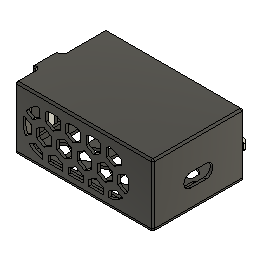
ESP32Case (Autodesk Fusion 360 design; units mm, degrees)
Autodesk Fusion 360 part; units mm, degrees
(part 1 of 3)
sketch "Skizze1" plane through (0, 0, 0) normal (0, 0, 1) x (1, 0, 0)
  line L0 (0, 0) -> (72, 0)
  line L1 (72, 0) -> (72, 49.5)
  line L2 (72, 49.5) -> (0, 49.5)
  line L3 (0, 49.5) -> (0, 0)
  dimension "d1" = 72
  dimension "d2" = 49.5
  constraint horizontal L0
  constraint vertical L1
  constraint horizontal L2
  constraint vertical L3
  constraint coincident L0.start L3.end
  measures "d1" distance of L0.start L0.end
  measures "d2" distance of L0.start L2.end
extrude "Extrusion1" add sketch "Skizze1" along normal blind 1.4 makes body 1
sketch "Skizze2" plane through (0, 0, 0) normal (0, 0, -1) x (1, 0, 0)
  line L0 (0, 0) -> (0, -49.5)
  line L1 (0, -49.5) -> (72, -49.5)
  line L2 (72, -49.5) -> (72, 0)
  line L3 (72, 0) -> (0, 0)
  line L4 (-2, -51.5) -> (74, -51.5)
  line L5 (74, -51.5) -> (74, 2)
  line L6 (74, 2) -> (-2, 2)
  line L7 (-2, 2) -> (-2, -51.5)
  line L8 (0, 0) -> (72, 0)
  line L9 (72, 0) -> (72, -4)
  line L10 (72, -4) -> (0, -4)
  line L11 (0, -4) -> (0, 0)
  line L12 (0, -49.5) -> (72, -49.5)
  line L13 (72, -49.5) -> (72, -45.5)
  line L14 (72, -45.5) -> (0, -45.5)
  line L15 (0, -45.5) -> (0, -49.5)
  line L16 (0, -49.5) -> (19, -49.5)
  line L17 (19, -49.5) -> (19, -45.5)
  line L18 (19, -45.5) -> (0, -45.5)
  line L19 (0, -45.5) -> (0, -49.5)
  line L20 (19, -45.5) -> (31, -45.5)
  line L21 (31, -45.5) -> (31, -49.5)
  line L22 (31, -49.5) -> (19, -49.5)
  line L23 (19, -49.5) -> (19, -45.5)
  line L24 (72, 0) -> (77, 0)
  line L25 (77, 0) -> (77, -49.5)
  line L26 (77, -49.5) -> (72, -49.5)
  line L27 (72, -49.5) -> (72, 0)
  line L28 (72, 2) -> (79, 2)
  line L29 (79, 2) -> (79, -51.5)
  line L30 (79, -51.5) -> (72, -51.5)
  dimension "d5" = 2
  dimension "d6" = 4
  dimension "d7" = 19
  dimension "d8" = 12
  dimension "d9" = 5
  dimension "d10" = -2
  constraint horizontal L8
  constraint vertical L9
  constraint horizontal L10
  constraint vertical L11
  constraint coincident L2 L9.end
  constraint coincident L0.start L3.end
  constraint horizontal L12
  constraint vertical L13
  constraint horizontal L14
  constraint vertical L15
  constraint coincident L0.end L1.start
  constraint horizontal L16
  constraint vertical L17
  constraint horizontal L18
  constraint vertical L19
  constraint horizontal L20
  constraint vertical L21
  constraint horizontal L22
  constraint vertical L23
  constraint horizontal L24
  constraint vertical L25
  constraint horizontal L26
  constraint vertical L27
  constraint coincident L2.end L3.start
  measures "d6" distance of L0.end L14.end
  measures "d7" distance of L0.end L16.end
  measures "d8" distance of L17.end L20.end
  measures "d9" distance of L2.end L24.end
extrude "Extrusion2" add sketch "Skizze2" along normal blind 2 separate body contours L0 L2 L3 L8 L9 L10 L11 L27 | L0 L1 L3 L4 L5 L6 L7 L8 L11 L12 L15 L16 L19 L22 L24 L26 L28 L30 | L2 L5 L9 L13 L24 L26 L27 | L0 L1 L12 L14 L15 L16 L17 L18 L19 L23 | L5 L24 L25 L26 | L5 L24 L25 L26 L28 L29 L30 | L1 L2 L12 L13 L14 L21 L27 makes body 2
sketch "Skizze3" plane through (0, 0, 0) normal (0, 0, 1) x (-1, 0, 0)
  line L0 (-72, -4) -> (0, -4)
  line L1 (0, -4) -> (0, -45.5)
  line L2 (0, -45.5) -> (-19, -45.5)
  line L3 (-19, -45.5) -> (-19, -49.5)
  line L4 (-19, -49.5) -> (-31, -49.5)
  line L5 (-31, -49.5) -> (-31, -45.5)
  line L6 (-31, -45.5) -> (-72, -45.5)
  line L7 (-72, -45.5) -> (-72, -4)
  line L8 (2, 2) -> (-79, 2)
  line L9 (-79, 2) -> (-79, -51.5)
  line L10 (-79, -51.5) -> (2, -51.5)
  line L11 (2, -51.5) -> (2, 2)
extrude "Extrusion3" add sketch "Skizze3" along normal blind 2 contours L0 L1 L2 L3 L4 L5 L6 L7 | L8 L9 L10 L11 bodies 2
move_body "Verschieben1" bodies 1 to x (1, 0, 0) y (0, 1, 0) z (0, 0, 1) at (0, 0, -3.4)
sketch "Skizze4" plane through (0, 0, -2) normal (0, 0, -1) x (1, 0, 0)
  line L0 (0, -4) -> (72, -4)
  line L1 (72, -4) -> (72, -45.5)
  line L2 (72, -45.5) -> (31, -45.5)
  line L3 (31, -45.5) -> (31, -49.5)
  line L4 (31, -49.5) -> (19, -49.5)
  line L5 (19, -49.5) -> (19, -45.5)
  line L6 (19, -45.5) -> (0, -45.5)
  line L7 (0, -45.5) -> (0, -4)
  line L8 (79, 2) -> (-2, 2)
  line L9 (-2, 2) -> (-2, -51.5)
  line L10 (-2, -51.5) -> (79, -51.5)
  line L11 (79, -51.5) -> (79, 2)
  line L12 (-0.5, -50) -> (77.5, -50)
  line L13 (77.5, -50) -> (77.5, 0.5)
  line L14 (77.5, 0.5) -> (-0.5, 0.5)
  line L15 (-0.5, 0.5) -> (-0.5, -50)
  line L16 (72, -4) -> (72, 0.5)
  line L17 (72, -45.5) -> (72, -50)
  line L18 (72, 0.5) -> (73.5, 0.5)
  line L19 (73.5, 0.5) -> (73.5, -50)
  line L20 (73.5, -50) -> (72, -50)
  line L21 (72, -50) -> (72, 0.5)
  dimension "d15" = -1.5
  dimension "d16" = 1.5
  constraint coincident L0.end L1.start
  constraint coincident L14 L16.end
  constraint perpendicular L14 L16
  constraint coincident L1.end L2.start
  constraint coincident L12 L17.end
  constraint perpendicular L12 L17
  constraint horizontal L18
  constraint vertical L19
  constraint horizontal L20
  constraint vertical L21
  measures "d16" distance of L16.end L18.end
extrude "Extrusion4" add sketch "Skizze4" along normal blind 31 bodies 2
extrude "Extrusion5" add sketch "Skizze4" along normal blind 12.4 contours L1 L12 L14 L16 L17 L18 L19 L20 L21 bodies 2
extrude "Extrusion6" add sketch "Skizze4" along normal blind 12.4 contours L12 L13 L14 L19 bodies 2
sketch "Skizze5" plane through (0, 0, -33) normal (0, 0, -1) x (1, 0, 0)
  line L0 (77.5, 0.5) -> (77.5, -50)
  line L1 (77.5, -50) -> (-0.5, -50)
  line L2 (-0.5, -50) -> (-0.5, 0.5)
  line L3 (-0.5, 0.5) -> (77.5, 0.5)
  line L4 (79, -51.5) -> (79, 2)
  line L5 (79, 2) -> (-2, 2)
  line L6 (-2, 2) -> (-2, -51.5)
  line L7 (-2, -51.5) -> (79, -51.5)
  line L8 (-2, -15.5) -> (7, -15.5)
  line L9 (0, 0) -> (72, 0)
  line L10 (-2, -21.5) -> (2, -21.5)
  line L11 (-2, -15.5) -> (0, -15.5)
  line L12 (0, -15.5) -> (0, -21.5)
  line L13 (0, -21.5) -> (-2, -21.5)
  line L14 (-2, -21.5) -> (-2, -15.5)
  dimension "d23" = 15.5
  dimension "d24" = 6
  constraint coincident L6 L8.start
  constraint perpendicular L6 L8
  constraint coincident L6 L10.start
  constraint perpendicular L2 L10
  constraint horizontal L11
  constraint vertical L12
  constraint horizontal L13
  constraint vertical L14
  constraint midpoint L10 L12.end
  measures "d23" distance of L8 L9
  measures "d24" distance of L8 L10
extrude "Extrusion7" cut sketch "Skizze5" against normal blind 27 contours L2 L6 L8 L10 L11 L13 L14 bodies 2
sketch "Skizze6" plane through (-2, 0, 0) normal (-1, 0, 0) x (0, -1, 0)
  line L0 (-15.5, -6) -> (-15.5, -33)
  line L1 (-15.5, -33) -> (2, -33)
  line L2 (2, -33) -> (2, 2)
  line L3 (2, 2) -> (-51.5, 2)
  line L4 (-51.5, 2) -> (-51.5, -33)
  line L5 (-51.5, -33) -> (-21.5, -33)
  line L6 (-21.5, -33) -> (-21.5, -6)
  line L7 (-21.5, -6) -> (-15.5, -6)
  line L8 (0, -3.4) -> (-49.5, -3.4)
  line L9 (-49.5, -3.4) -> (0, -3.4)
  circle A0 centre (-18.5, -6.4) radius 3
  constraint tangent L8 A0
  constraint tangent L0 A0
  constraint tangent L6 A0
extrude "Extrusion8" cut sketch "Skizze6" against normal blind 1.5 contours L7 A0 picked at (-17.8417, -5.3806) bodies 2
sketch "Skizze7" plane through (79, 0, 0) normal (1, 0, 0) x (0, 1, 0)
  line L0 (-2, 2) -> (-2, -33)
  line L1 (-2, -33) -> (51.5, -33)
  line L2 (51.5, -33) -> (51.5, 2)
  line L3 (51.5, 2) -> (-2, 2)
  line L4 (50, -14.4) -> (-0.5, -14.4)
  line L5 (-0.5, -14.4) -> (50, -14.4)
  line L6 (48.75, -19) -> (0.75, -19) construction
  line L7 (29.25, -15) -> (20.25, -15)
  arc A0 (20.25, -15) -> (20.25, -23) centre (20.25, -19) ccw
  line L8 (20.25, -23) -> (29.25, -23)
  arc A1 (29.25, -23) -> (29.25, -15) centre (29.25, -19) ccw
  line L9 (29.25, -19) -> (20.25, -19) construction
  point P0 (24.75, -19)
  dimension "d29" = 4.6
  dimension "d30" = 8
  dimension "d31" = 9
  dimension "d32" = 53.5
  dimension "d33" = 26.75
  constraint parallel L4 L6
  constraint tangent L7 A0
  constraint tangent A0 L8
  constraint parallel L7 L8
  constraint tangent L8 A1
  constraint tangent L7 A1
  constraint parallel L6 L9
  constraint midpoint L6 P0
  constraint midpoint L9 P0
  measures "d29" distance of L4 L6
  measures "d30" diameter of A0
  measures "d31" distance of A0.end L8.end
  measures "d32" distance of L0.end L1.end
  measures "d33" distance of L0 P0
extrude "Extrusion9" cut sketch "Skizze7" against normal blind 7 contours L7 A0 L8 A1 bodies 2
sketch "Skizze8" plane through (0, 51.5, 0) normal (0, 1, 0) x (-1, 0, 0)
  line L0 (-79, 2) -> (-79, -33)
  line L1 (-79, -33) -> (2, -33)
  line L2 (2, -33) -> (2, 2)
  line L3 (2, 2) -> (-79, 2)
  line L4 (-72, -14.4) -> (-77.5, -14.4)
  line L5 (-77.5, -15) -> (-79, -15)
  line L6 (-79, -15) -> (-77.5, -15)
  line L7 (-77.5, -14.4) -> (-72, -14.4)
  line L8 (-77.5, -14.4) -> (-70, -14.4)
  line L9 (-70, -14.4) -> (-70, -16)
  line L10 (-70, -16) -> (-77.5, -16)
  line L11 (-77.5, -16) -> (-77.5, -14.4)
  line L12 (-77.5, -16) -> (-71.5, -16)
  line L13 (-71.5, -16) -> (-71.5, -20)
  line L14 (-71.5, -20) -> (-77.5, -20)
  line L15 (-77.5, -20) -> (-77.5, -16)
  line L16 (-79, -14.5) -> (-70, -14.5)
  line L17 (-70, -14.5) -> (-70, -21.5)
  line L18 (-70, -21.5) -> (-79, -21.5)
  line L19 (-79, -21.5) -> (-79, -14.5)
  dimension "d36" = 6
  dimension "d37" = 4
  dimension "d38" = -1.5
  constraint horizontal L8
  constraint vertical L9
  constraint horizontal L10
  constraint vertical L11
  constraint coincident L4.end L7.start
  constraint horizontal L12
  constraint vertical L13
  constraint horizontal L14
  constraint vertical L15
  measures "d36" distance of L10.end L12.end
  measures "d37" distance of L10.end L14.end
extrude "Extrusion10" add sketch "Skizze8" against normal blind 8 contours L0 L5 L6 L11 L16 L19 | L0 L5 L6 L10 L11 L13 L14 L15 L17 L18 L19 | L9 L10 L11 L12 L16 L17 bodies 2
extrude "Extrusion11" add 1 faces at (75, 45.6667, -14.5) along direction (0, 0, 1) blind 0.1 on bodies 2 bodies 2
chamfer "Fase1" distance 2 angle 45 1 edges at (72, 46.75, -14.4) on bodies 2
extrude "Extrusion12" cut 1 faces at (73.5, 50, -18.6667) along direction (0, 1, 0) blind 10 on bodies 2 bodies 2
sketch "Skizze9" plane through (0, 51.5, 0) normal (0, 1, 0) x (-1, 0, 0)
  line L0 (-71.5, -16) -> (-71.5, -20)
  line L1 (-71.5, -20) -> (-77.5, -20)
  line L2 (-77.5, -20) -> (-77.5, -16)
  line L3 (-77.5, -16) -> (-71.5, -16)
  line L4 (-79, 2) -> (-79, -33)
  line L5 (-79, -33) -> (2, -33)
  line L6 (2, -33) -> (2, 2)
  line L7 (2, 2) -> (-79, 2)
  line L8 (-51.9385, -29.7827) -> (-15.9385, -29.7827)
  arc A0 (-15.9385, -29.7827) -> (-15.9385, -3.6265) centre (-15.9385, -16.7046) ccw
  line L9 (-15.9385, -3.6265) -> (-51.9385, -3.6265)
  arc A1 (-51.9385, -3.6265) -> (-51.9385, -29.7827) centre (-51.9385, -16.7046) ccw
  line L10 (-51.9385, -16.7046) -> (-15.9385, -16.7046) construction
  line L11 (0, -3.4) -> (-72, -3.4)
  line L12 (-72, -3.4) -> (0, -3.4)
  line L13 (106.9565, 20) -> (111.2866, 22.5)
  line L14 (111.2866, 22.5) -> (111.2866, 27.5)
  line L15 (111.2866, 27.5) -> (106.9565, 30)
  line L16 (106.9565, 30) -> (102.6264, 27.5)
  line L17 (102.6264, 27.5) -> (102.6264, 22.5)
  line L18 (102.6264, 22.5) -> (106.9565, 20)
  line L19 (106.9565, 30) -> (34, 30)
  line L20 (99.3775, 22.5) -> (99.3775, 27.5)
  line L21 (99.3775, 27.5) -> (95.0474, 30)
  line L22 (95.0474, 30) -> (90.7173, 27.5)
  line L23 (90.7173, 27.5) -> (90.7173, 22.5)
  line L24 (90.7173, 22.5) -> (95.0474, 20)
  line L25 (95.0474, 20) -> (99.3775, 22.5)
  line L26 (87.4684, 22.5) -> (87.4684, 27.5)
  line L27 (87.4684, 27.5) -> (83.1383, 30)
  line L28 (83.1383, 30) -> (78.8082, 27.5)
  line L29 (78.8082, 27.5) -> (78.8082, 22.5)
  line L30 (78.8082, 22.5) -> (83.1383, 20)
  line L31 (83.1383, 20) -> (87.4684, 22.5)
  line L32 (75.5593, 22.5) -> (75.5593, 27.5)
  line L33 (75.5593, 27.5) -> (71.2292, 30)
  line L34 (71.2292, 30) -> (66.8991, 27.5)
  line L35 (66.8991, 27.5) -> (66.8991, 22.5)
  line L36 (66.8991, 22.5) -> (71.2292, 20)
  line L37 (71.2292, 20) -> (75.5593, 22.5)
  line L38 (63.6503, 22.5) -> (63.6503, 27.5)
  line L39 (63.6503, 27.5) -> (59.3201, 30)
  line L40 (59.3201, 30) -> (54.99, 27.5)
  line L41 (54.99, 27.5) -> (54.99, 22.5)
  line L42 (54.99, 22.5) -> (59.3201, 20)
  line L43 (59.3201, 20) -> (63.6503, 22.5)
  line L44 (51.7412, 22.5) -> (51.7412, 27.5)
  line L45 (51.7412, 27.5) -> (47.411, 30)
  line L46 (47.411, 30) -> (43.0809, 27.5)
  line L47 (43.0809, 27.5) -> (43.0809, 22.5)
  line L48 (43.0809, 22.5) -> (47.411, 20)
  line L49 (47.411, 20) -> (51.7412, 22.5)
  line L50 (39.8321, 22.5) -> (39.8321, 27.5)
  line L51 (39.8321, 27.5) -> (35.5019, 30)
  line L52 (35.5019, 30) -> (31.1718, 27.5)
  line L53 (31.1718, 27.5) -> (31.1718, 22.5)
  line L54 (31.1718, 22.5) -> (35.5019, 20)
  line L55 (35.5019, 20) -> (39.8321, 22.5)
  line L56 (27.923, 22.5) -> (27.923, 27.5)
  line L57 (27.923, 27.5) -> (23.5929, 30)
  line L58 (23.5929, 30) -> (19.2627, 27.5)
  line L59 (19.2627, 27.5) -> (19.2627, 22.5)
  line L60 (19.2627, 22.5) -> (23.5929, 20)
  line L61 (23.5929, 20) -> (27.923, 22.5)
  line L62 (16.0139, 22.5) -> (16.0139, 27.5)
  line L63 (16.0139, 27.5) -> (11.6838, 30)
  line L64 (11.6838, 30) -> (7.3536, 27.5)
  line L65 (7.3536, 27.5) -> (7.3536, 22.5)
  line L66 (7.3536, 22.5) -> (11.6838, 20)
  line L67 (11.6838, 20) -> (16.0139, 22.5)
  line L68 (4.1048, 22.5) -> (4.1048, 27.5)
  line L69 (4.1048, 27.5) -> (-0.2253, 30)
  line L70 (-0.2253, 30) -> (-4.5555, 27.5)
  line L71 (-4.5555, 27.5) -> (-4.5555, 22.5)
  line L72 (-4.5555, 22.5) -> (-0.2253, 20)
  line L73 (-0.2253, 20) -> (4.1048, 22.5)
  line L74 (-7.8043, 22.5) -> (-7.8043, 27.5)
  line L75 (-7.8043, 27.5) -> (-12.1344, 30)
  line L76 (-12.1344, 30) -> (-16.4645, 27.5)
  line L77 (-16.4645, 27.5) -> (-16.4645, 22.5)
  line L78 (-16.4645, 22.5) -> (-12.1344, 20)
  line L79 (-12.1344, 20) -> (-7.8043, 22.5)
  line L80 (-19.7134, 22.5) -> (-19.7134, 27.5)
  line L81 (-19.7134, 27.5) -> (-24.0435, 30)
  line L82 (-24.0435, 30) -> (-28.3736, 27.5)
  line L83 (-28.3736, 27.5) -> (-28.3736, 22.5)
  line L84 (-28.3736, 22.5) -> (-24.0435, 20)
  line L85 (-24.0435, 20) -> (-19.7134, 22.5)
  line L86 (92.6671, 11.75) -> (92.6671, 16.75)
  line L87 (92.6671, 16.75) -> (88.3369, 19.25)
  line L88 (88.3369, 19.25) -> (84.0068, 16.75)
  line L89 (84.0068, 16.75) -> (84.0068, 11.75)
  line L90 (84.0068, 11.75) -> (88.3369, 9.25)
  line L91 (88.3369, 9.25) -> (92.6671, 11.75)
  line L92 (80.758, 11.75) -> (80.758, 16.75)
  line L93 (80.758, 16.75) -> (76.4279, 19.25)
  line L94 (76.4279, 19.25) -> (72.0977, 16.75)
  line L95 (72.0977, 16.75) -> (72.0977, 11.75)
  line L96 (72.0977, 11.75) -> (76.4279, 9.25)
  line L97 (76.4279, 9.25) -> (80.758, 11.75)
  line L98 (68.8489, 11.75) -> (68.8489, 16.75)
  line L99 (68.8489, 16.75) -> (64.5188, 19.25)
  line L100 (64.5188, 19.25) -> (60.1886, 16.75)
  line L101 (60.1886, 16.75) -> (60.1886, 11.75)
  line L102 (60.1886, 11.75) -> (64.5188, 9.25)
  line L103 (64.5188, 9.25) -> (68.8489, 11.75)
  line L104 (56.9398, 11.75) -> (56.9398, 16.75)
  line L105 (56.9398, 16.75) -> (52.6097, 19.25)
  line L106 (52.6097, 19.25) -> (48.2795, 16.75)
  line L107 (48.2795, 16.75) -> (48.2795, 11.75)
  line L108 (48.2795, 11.75) -> (52.6097, 9.25)
  line L109 (52.6097, 9.25) -> (56.9398, 11.75)
  line L110 (45.0307, 11.75) -> (45.0307, 16.75)
  line L111 (45.0307, 16.75) -> (40.7006, 19.25)
  line L112 (40.7006, 19.25) -> (36.3705, 16.75)
  line L113 (36.3705, 16.75) -> (36.3705, 11.75)
  line L114 (36.3705, 11.75) -> (40.7006, 9.25)
  line L115 (40.7006, 9.25) -> (45.0307, 11.75)
  line L116 (33.1216, 11.75) -> (33.1216, 16.75)
  line L117 (33.1216, 16.75) -> (28.7915, 19.25)
  line L118 (28.7915, 19.25) -> (24.4614, 16.75)
  line L119 (24.4614, 16.75) -> (24.4614, 11.75)
  line L120 (24.4614, 11.75) -> (28.7915, 9.25)
  line L121 (28.7915, 9.25) -> (33.1216, 11.75)
  line L122 (21.2125, 11.75) -> (21.2125, 16.75)
  line L123 (21.2125, 16.75) -> (16.8824, 19.25)
  line L124 (16.8824, 19.25) -> (12.5523, 16.75)
  line L125 (12.5523, 16.75) -> (12.5523, 11.75)
  line L126 (12.5523, 11.75) -> (16.8824, 9.25)
  line L127 (16.8824, 9.25) -> (21.2125, 11.75)
  line L128 (9.3034, 11.75) -> (9.3034, 16.75)
  line L129 (9.3034, 16.75) -> (4.9733, 19.25)
  line L130 (4.9733, 19.25) -> (0.6432, 16.75)
  line L131 (0.6432, 16.75) -> (0.6432, 11.75)
  line L132 (0.6432, 11.75) -> (4.9733, 9.25)
  line L133 (4.9733, 9.25) -> (9.3034, 11.75)
  line L134 (-2.6057, 11.75) -> (-2.6057, 16.75)
  line L135 (-2.6057, 16.75) -> (-6.9358, 19.25)
  line L136 (-6.9358, 19.25) -> (-11.2659, 16.75)
  line L137 (-11.2659, 16.75) -> (-11.2659, 11.75)
  line L138 (-11.2659, 11.75) -> (-6.9358, 9.25)
  line L139 (-6.9358, 9.25) -> (-2.6057, 11.75)
  line L140 (-14.5147, 11.75) -> (-14.5147, 16.75)
  line L141 (-14.5147, 16.75) -> (-18.8449, 19.25)
  line L142 (-18.8449, 19.25) -> (-23.175, 16.75)
  line L143 (-23.175, 16.75) -> (-23.175, 11.75)
  line L144 (-23.175, 11.75) -> (-18.8449, 9.25)
  line L145 (-18.8449, 9.25) -> (-14.5147, 11.75)
  line L146 (-26.4238, 11.75) -> (-26.4238, 16.75)
  line L147 (-26.4238, 16.75) -> (-30.754, 19.25)
  line L148 (-30.754, 19.25) -> (-35.0841, 16.75)
  line L149 (-35.0841, 16.75) -> (-35.0841, 11.75)
  line L150 (-35.0841, 11.75) -> (-30.754, 9.25)
  line L151 (-30.754, 9.25) -> (-26.4238, 11.75)
  line L152 (-38.3329, 11.75) -> (-38.3329, 16.75)
  line L153 (-38.3329, 16.75) -> (-42.6631, 19.25)
  line L154 (-42.6631, 19.25) -> (-46.9932, 16.75)
  line L155 (-46.9932, 16.75) -> (-46.9932, 11.75)
  line L156 (-46.9932, 11.75) -> (-42.6631, 9.25)
  line L157 (-42.6631, 9.25) -> (-38.3329, 11.75)
  line L158 (74.0475, 1) -> (74.0475, 6)
  line L159 (74.0475, 6) -> (69.7174, 8.5)
  line L160 (69.7174, 8.5) -> (65.3873, 6)
  line L161 (65.3873, 6) -> (65.3873, 1)
  line L162 (65.3873, 1) -> (69.7174, -1.5)
  line L163 (69.7174, -1.5) -> (74.0475, 1)
  line L164 (62.1384, 1) -> (62.1384, 6)
  line L165 (62.1384, 6) -> (57.8083, 8.5)
  line L166 (57.8083, 8.5) -> (53.4782, 6)
  line L167 (53.4782, 6) -> (53.4782, 1)
  line L168 (53.4782, 1) -> (57.8083, -1.5)
  line L169 (57.8083, -1.5) -> (62.1384, 1)
  line L170 (50.2293, 1) -> (50.2293, 6)
  line L171 (50.2293, 6) -> (45.8992, 8.5)
  line L172 (45.8992, 8.5) -> (41.5691, 6)
  line L173 (41.5691, 6) -> (41.5691, 1)
  line L174 (41.5691, 1) -> (45.8992, -1.5)
  line L175 (45.8992, -1.5) -> (50.2293, 1)
  line L176 (38.3203, 1) -> (38.3203, 6)
  line L177 (38.3203, 6) -> (33.9901, 8.5)
  line L178 (33.9901, 8.5) -> (29.66, 6)
  line L179 (29.66, 6) -> (29.66, 1)
  line L180 (29.66, 1) -> (33.9901, -1.5)
  line L181 (33.9901, -1.5) -> (38.3203, 1)
  line L182 (26.4112, 1) -> (26.4112, 6)
  line L183 (26.4112, 6) -> (22.081, 8.5)
  line L184 (22.081, 8.5) -> (17.7509, 6)
  line L185 (17.7509, 6) -> (17.7509, 1)
  line L186 (17.7509, 1) -> (22.081, -1.5)
  line L187 (22.081, -1.5) -> (26.4112, 1)
  line L188 (14.5021, 1) -> (14.5021, 6)
  line L189 (14.5021, 6) -> (10.1719, 8.5)
  line L190 (10.1719, 8.5) -> (5.8418, 6)
  line L191 (5.8418, 6) -> (5.8418, 1)
  line L192 (5.8418, 1) -> (10.1719, -1.5)
  line L193 (10.1719, -1.5) -> (14.5021, 1)
  line L194 (2.593, 1) -> (2.593, 6)
  line L195 (2.593, 6) -> (-1.7371, 8.5)
  line L196 (-1.7371, 8.5) -> (-6.0673, 6)
  line L197 (-6.0673, 6) -> (-6.0673, 1)
  line L198 (-6.0673, 1) -> (-1.7371, -1.5)
  line L199 (-1.7371, -1.5) -> (2.593, 1)
  line L200 (-9.3161, 1) -> (-9.3161, 6)
  line L201 (-9.3161, 6) -> (-13.6462, 8.5)
  line L202 (-13.6462, 8.5) -> (-17.9764, 6)
  line L203 (-17.9764, 6) -> (-17.9764, 1)
  line L204 (-17.9764, 1) -> (-13.6462, -1.5)
  line L205 (-13.6462, -1.5) -> (-9.3161, 1)
  line L206 (-21.2252, 1) -> (-21.2252, 6)
  line L207 (-21.2252, 6) -> (-25.5553, 8.5)
  line L208 (-25.5553, 8.5) -> (-29.8855, 6)
  line L209 (-29.8855, 6) -> (-29.8855, 1)
  line L210 (-29.8855, 1) -> (-25.5553, -1.5)
  line L211 (-25.5553, -1.5) -> (-21.2252, 1)
  line L212 (-33.1343, 1) -> (-33.1343, 6)
  line L213 (-33.1343, 6) -> (-37.4644, 8.5)
  line L214 (-37.4644, 8.5) -> (-41.7945, 6)
  line L215 (-41.7945, 6) -> (-41.7945, 1)
  line L216 (-41.7945, 1) -> (-37.4644, -1.5)
  line L217 (-37.4644, -1.5) -> (-33.1343, 1)
  line L218 (-45.0434, 1) -> (-45.0434, 6)
  line L219 (-45.0434, 6) -> (-49.3735, 8.5)
  line L220 (-49.3735, 8.5) -> (-53.7036, 6)
  line L221 (-53.7036, 6) -> (-53.7036, 1)
  line L222 (-53.7036, 1) -> (-49.3735, -1.5)
  line L223 (-49.3735, -1.5) -> (-45.0434, 1)
  line L224 (-56.9525, 1) -> (-56.9525, 6)
  line L225 (-56.9525, 6) -> (-61.2826, 8.5)
  line L226 (-61.2826, 8.5) -> (-65.6127, 6)
  line L227 (-65.6127, 6) -> (-65.6127, 1)
  line L228 (-65.6127, 1) -> (-61.2826, -1.5)
  line L229 (-61.2826, -1.5) -> (-56.9525, 1)
  line L230 (55.428, -9.75) -> (55.428, -4.75)
  line L231 (55.428, -4.75) -> (51.0979, -2.25)
  line L232 (51.0979, -2.25) -> (46.7677, -4.75)
  line L233 (46.7677, -4.75) -> (46.7677, -9.75)
  line L234 (46.7677, -9.75) -> (51.0979, -12.25)
  line L235 (51.0979, -12.25) -> (55.428, -9.75)
  line L236 (43.5189, -9.75) -> (43.5189, -4.75)
  line L237 (43.5189, -4.75) -> (39.1888, -2.25)
  line L238 (39.1888, -2.25) -> (34.8586, -4.75)
  line L239 (34.8586, -4.75) -> (34.8586, -9.75)
  line L240 (34.8586, -9.75) -> (39.1888, -12.25)
  line L241 (39.1888, -12.25) -> (43.5189, -9.75)
  line L242 (31.6098, -9.75) -> (31.6098, -4.75)
  line L243 (31.6098, -4.75) -> (27.2797, -2.25)
  line L244 (27.2797, -2.25) -> (22.9495, -4.75)
  line L245 (22.9495, -4.75) -> (22.9495, -9.75)
  line L246 (22.9495, -9.75) -> (27.2797, -12.25)
  line L247 (27.2797, -12.25) -> (31.6098, -9.75)
  line L248 (19.7007, -9.75) -> (19.7007, -4.75)
  line L249 (19.7007, -4.75) -> (15.3706, -2.25)
  line L250 (15.3706, -2.25) -> (11.0405, -4.75)
  line L251 (11.0405, -4.75) -> (11.0405, -9.75)
  line L252 (11.0405, -9.75) -> (15.3706, -12.25)
  line L253 (15.3706, -12.25) -> (19.7007, -9.75)
  line L254 (7.7916, -9.75) -> (7.7916, -4.75)
  line L255 (7.7916, -4.75) -> (3.4615, -2.25)
  line L256 (3.4615, -2.25) -> (-0.8686, -4.75)
  line L257 (-0.8686, -4.75) -> (-0.8686, -9.75)
  line L258 (-0.8686, -9.75) -> (3.4615, -12.25)
  line L259 (3.4615, -12.25) -> (7.7916, -9.75)
  line L260 (-4.1175, -9.75) -> (-4.1175, -4.75)
  line L261 (-4.1175, -4.75) -> (-8.4476, -2.25)
  line L262 (-8.4476, -2.25) -> (-12.7777, -4.75)
  line L263 (-12.7777, -4.75) -> (-12.7777, -9.75)
  line L264 (-12.7777, -9.75) -> (-8.4476, -12.25)
  line L265 (-8.4476, -12.25) -> (-4.1175, -9.75)
  line L266 (-16.0266, -9.75) -> (-16.0266, -4.75)
  line L267 (-16.0266, -4.75) -> (-20.3567, -2.25)
  line L268 (-20.3567, -2.25) -> (-24.6868, -4.75)
  line L269 (-24.6868, -4.75) -> (-24.6868, -9.75)
  line L270 (-24.6868, -9.75) -> (-20.3567, -12.25)
  line L271 (-20.3567, -12.25) -> (-16.0266, -9.75)
  line L272 (-27.9357, -9.75) -> (-27.9357, -4.75)
  line L273 (-27.9357, -4.75) -> (-32.2658, -2.25)
  line L274 (-32.2658, -2.25) -> (-36.5959, -4.75)
  line L275 (-36.5959, -4.75) -> (-36.5959, -9.75)
  line L276 (-36.5959, -9.75) -> (-32.2658, -12.25)
  line L277 (-32.2658, -12.25) -> (-27.9357, -9.75)
  line L278 (-39.8447, -9.75) -> (-39.8447, -4.75)
  line L279 (-39.8447, -4.75) -> (-44.1749, -2.25)
  line L280 (-44.1749, -2.25) -> (-48.505, -4.75)
  line L281 (-48.505, -4.75) -> (-48.505, -9.75)
  line L282 (-48.505, -9.75) -> (-44.1749, -12.25)
  line L283 (-44.1749, -12.25) -> (-39.8447, -9.75)
  line L284 (-51.7538, -9.75) -> (-51.7538, -4.75)
  line L285 (-51.7538, -4.75) -> (-56.084, -2.25)
  line L286 (-56.084, -2.25) -> (-60.4141, -4.75)
  line L287 (-60.4141, -4.75) -> (-60.4141, -9.75)
  line L288 (-60.4141, -9.75) -> (-56.084, -12.25)
  line L289 (-56.084, -12.25) -> (-51.7538, -9.75)
  line L290 (-63.6629, -9.75) -> (-63.6629, -4.75)
  line L291 (-63.6629, -4.75) -> (-67.9931, -2.25)
  line L292 (-67.9931, -2.25) -> (-72.3232, -4.75)
  line L293 (-72.3232, -4.75) -> (-72.3232, -9.75)
  line L294 (-72.3232, -9.75) -> (-67.9931, -12.25)
  line L295 (-67.9931, -12.25) -> (-63.6629, -9.75)
  line L296 (-75.572, -9.75) -> (-75.572, -4.75)
  line L297 (-75.572, -4.75) -> (-79.9021, -2.25)
  line L298 (-79.9021, -2.25) -> (-84.2323, -4.75)
  line L299 (-84.2323, -4.75) -> (-84.2323, -9.75)
  line L300 (-84.2323, -9.75) -> (-79.9021, -12.25)
  line L301 (-79.9021, -12.25) -> (-75.572, -9.75)
  line L302 (36.8084, -20.5) -> (36.8084, -15.5)
  line L303 (36.8084, -15.5) -> (32.4783, -13)
  line L304 (32.4783, -13) -> (28.1482, -15.5)
  line L305 (28.1482, -15.5) -> (28.1482, -20.5)
  line L306 (28.1482, -20.5) -> (32.4783, -23)
  line L307 (32.4783, -23) -> (36.8084, -20.5)
  line L308 (24.8993, -20.5) -> (24.8993, -15.5)
  line L309 (24.8993, -15.5) -> (20.5692, -13)
  line L310 (20.5692, -13) -> (16.2391, -15.5)
  line L311 (16.2391, -15.5) -> (16.2391, -20.5)
  line L312 (16.2391, -20.5) -> (20.5692, -23)
  line L313 (20.5692, -23) -> (24.8993, -20.5)
  line L314 (12.9902, -20.5) -> (12.9902, -15.5)
  line L315 (12.9902, -15.5) -> (8.6601, -13)
  line L316 (8.6601, -13) -> (4.33, -15.5)
  line L317 (4.33, -15.5) -> (4.33, -20.5)
  line L318 (4.33, -20.5) -> (8.6601, -23)
  line L319 (8.6601, -23) -> (12.9902, -20.5)
  line L320 (1.0812, -20.5) -> (1.0812, -15.5)
  line L321 (1.0812, -15.5) -> (-3.249, -13)
  line L322 (-3.249, -13) -> (-7.5791, -15.5)
  line L323 (-7.5791, -15.5) -> (-7.5791, -20.5)
  line L324 (-7.5791, -20.5) -> (-3.249, -23)
  line L325 (-3.249, -23) -> (1.0812, -20.5)
  line L326 (-10.8279, -20.5) -> (-10.8279, -15.5)
  line L327 (-10.8279, -15.5) -> (-15.1581, -13)
  line L328 (-15.1581, -13) -> (-19.4882, -15.5)
  line L329 (-19.4882, -15.5) -> (-19.4882, -20.5)
  line L330 (-19.4882, -20.5) -> (-15.1581, -23)
  line L331 (-15.1581, -23) -> (-10.8279, -20.5)
  line L332 (-22.737, -20.5) -> (-22.737, -15.5)
  line L333 (-22.737, -15.5) -> (-27.0672, -13)
  line L334 (-27.0672, -13) -> (-31.3973, -15.5)
  line L335 (-31.3973, -15.5) -> (-31.3973, -20.5)
  line L336 (-31.3973, -20.5) -> (-27.0672, -23)
  line L337 (-27.0672, -23) -> (-22.737, -20.5)
  line L338 (-34.6461, -20.5) -> (-34.6461, -15.5)
  line L339 (-34.6461, -15.5) -> (-38.9762, -13)
  line L340 (-38.9762, -13) -> (-43.3064, -15.5)
  line L341 (-43.3064, -15.5) -> (-43.3064, -20.5)
  line L342 (-43.3064, -20.5) -> (-38.9762, -23)
  line L343 (-38.9762, -23) -> (-34.6461, -20.5)
  line L344 (-46.5552, -20.5) -> (-46.5552, -15.5)
  line L345 (-46.5552, -15.5) -> (-50.8853, -13)
  line L346 (-50.8853, -13) -> (-55.2155, -15.5)
  line L347 (-55.2155, -15.5) -> (-55.2155, -20.5)
  line L348 (-55.2155, -20.5) -> (-50.8853, -23)
  line L349 (-50.8853, -23) -> (-46.5552, -20.5)
  line L350 (-58.4643, -20.5) -> (-58.4643, -15.5)
  line L351 (-58.4643, -15.5) -> (-62.7944, -13)
  line L352 (-62.7944, -13) -> (-67.1245, -15.5)
  line L353 (-67.1245, -15.5) -> (-67.1245, -20.5)
  line L354 (-67.1245, -20.5) -> (-62.7944, -23)
  line L355 (-62.7944, -23) -> (-58.4643, -20.5)
  line L356 (-70.3734, -20.5) -> (-70.3734, -15.5)
  line L357 (-70.3734, -15.5) -> (-74.7035, -13)
  line L358 (-74.7035, -13) -> (-79.0336, -15.5)
  line L359 (-79.0336, -15.5) -> (-79.0336, -20.5)
  line L360 (-79.0336, -20.5) -> (-74.7035, -23)
  line L361 (-74.7035, -23) -> (-70.3734, -20.5)
  line L362 (-82.2825, -20.5) -> (-82.2825, -15.5)
  line L363 (-82.2825, -15.5) -> (-86.6126, -13)
  line L364 (-86.6126, -13) -> (-90.9427, -15.5)
  line L365 (-90.9427, -15.5) -> (-90.9427, -20.5)
  line L366 (-90.9427, -20.5) -> (-86.6126, -23)
  line L367 (-86.6126, -23) -> (-82.2825, -20.5)
  line L368 (-94.1916, -20.5) -> (-94.1916, -15.5)
  line L369 (-94.1916, -15.5) -> (-98.5217, -13)
  line L370 (-98.5217, -13) -> (-102.8518, -15.5)
  line L371 (-102.8518, -15.5) -> (-102.8518, -20.5)
  line L372 (-102.8518, -20.5) -> (-98.5217, -23)
  line L373 (-98.5217, -23) -> (-94.1916, -20.5)
  line L374 (18.1889, -31.25) -> (18.1889, -26.25)
  line L375 (18.1889, -26.25) -> (13.8588, -23.75)
  line L376 (13.8588, -23.75) -> (9.5286, -26.25)
  line L377 (9.5286, -26.25) -> (9.5286, -31.25)
  line L378 (9.5286, -31.25) -> (13.8588, -33.75)
  line L379 (13.8588, -33.75) -> (18.1889, -31.25)
  line L380 (6.2798, -31.25) -> (6.2798, -26.25)
  line L381 (6.2798, -26.25) -> (1.9497, -23.75)
  line L382 (1.9497, -23.75) -> (-2.3805, -26.25)
  line L383 (-2.3805, -26.25) -> (-2.3805, -31.25)
  line L384 (-2.3805, -31.25) -> (1.9497, -33.75)
  line L385 (1.9497, -33.75) -> (6.2798, -31.25)
  line L386 (-5.6293, -31.25) -> (-5.6293, -26.25)
  line L387 (-5.6293, -26.25) -> (-9.9594, -23.75)
  line L388 (-9.9594, -23.75) -> (-14.2896, -26.25)
  line L389 (-14.2896, -26.25) -> (-14.2896, -31.25)
  line L390 (-14.2896, -31.25) -> (-9.9594, -33.75)
  line L391 (-9.9594, -33.75) -> (-5.6293, -31.25)
  line L392 (-17.5384, -31.25) -> (-17.5384, -26.25)
  line L393 (-17.5384, -26.25) -> (-21.8685, -23.75)
  line L394 (-21.8685, -23.75) -> (-26.1986, -26.25)
  line L395 (-26.1986, -26.25) -> (-26.1986, -31.25)
  line L396 (-26.1986, -31.25) -> (-21.8685, -33.75)
  line L397 (-21.8685, -33.75) -> (-17.5384, -31.25)
  line L398 (-29.4475, -31.25) -> (-29.4475, -26.25)
  line L399 (-29.4475, -26.25) -> (-33.7776, -23.75)
  line L400 (-33.7776, -23.75) -> (-38.1077, -26.25)
  line L401 (-38.1077, -26.25) -> (-38.1077, -31.25)
  line L402 (-38.1077, -31.25) -> (-33.7776, -33.75)
  line L403 (-33.7776, -33.75) -> (-29.4475, -31.25)
  line L404 (-41.3566, -31.25) -> (-41.3566, -26.25)
  line L405 (-41.3566, -26.25) -> (-45.6867, -23.75)
  line L406 (-45.6867, -23.75) -> (-50.0168, -26.25)
  line L407 (-50.0168, -26.25) -> (-50.0168, -31.25)
  line L408 (-50.0168, -31.25) -> (-45.6867, -33.75)
  line L409 (-45.6867, -33.75) -> (-41.3566, -31.25)
  line L410 (-53.2657, -31.25) -> (-53.2657, -26.25)
  line L411 (-53.2657, -26.25) -> (-57.5958, -23.75)
  line L412 (-57.5958, -23.75) -> (-61.9259, -26.25)
  line L413 (-61.9259, -26.25) -> (-61.9259, -31.25)
  line L414 (-61.9259, -31.25) -> (-57.5958, -33.75)
  line L415 (-57.5958, -33.75) -> (-53.2657, -31.25)
  line L416 (-65.1748, -31.25) -> (-65.1748, -26.25)
  line L417 (-65.1748, -26.25) -> (-69.5049, -23.75)
  line L418 (-69.5049, -23.75) -> (-73.835, -26.25)
  line L419 (-73.835, -26.25) -> (-73.835, -31.25)
  line L420 (-73.835, -31.25) -> (-69.5049, -33.75)
  line L421 (-69.5049, -33.75) -> (-65.1748, -31.25)
  line L422 (-77.0838, -31.25) -> (-77.0838, -26.25)
  line L423 (-77.0838, -26.25) -> (-81.414, -23.75)
  line L424 (-81.414, -23.75) -> (-85.7441, -26.25)
  line L425 (-85.7441, -26.25) -> (-85.7441, -31.25)
  line L426 (-85.7441, -31.25) -> (-81.414, -33.75)
  line L427 (-81.414, -33.75) -> (-77.0838, -31.25)
  line L428 (-88.9929, -31.25) -> (-88.9929, -26.25)
  line L429 (-88.9929, -26.25) -> (-93.3231, -23.75)
  line L430 (-93.3231, -23.75) -> (-97.6532, -26.25)
  line L431 (-97.6532, -26.25) -> (-97.6532, -31.25)
  line L432 (-97.6532, -31.25) -> (-93.3231, -33.75)
  line L433 (-93.3231, -33.75) -> (-88.9929, -31.25)
  line L434 (-100.902, -31.25) -> (-100.902, -26.25)
  line L435 (-100.902, -26.25) -> (-105.2322, -23.75)
  line L436 (-105.2322, -23.75) -> (-109.5623, -26.25)
  line L437 (-109.5623, -26.25) -> (-109.5623, -31.25)
  line L438 (-109.5623, -31.25) -> (-105.2322, -33.75)
  line L439 (-105.2322, -33.75) -> (-100.902, -31.25)
  line L440 (-112.8111, -31.25) -> (-112.8111, -26.25)
  line L441 (-112.8111, -26.25) -> (-117.1412, -23.75)
  line L442 (-117.1412, -23.75) -> (-121.4714, -26.25)
  line L443 (-121.4714, -26.25) -> (-121.4714, -31.25)
  line L444 (-121.4714, -31.25) -> (-117.1412, -33.75)
  line L445 (-117.1412, -33.75) -> (-112.8111, -31.25)
  line L446 (-0.4307, -42) -> (-0.4307, -37)
  line L447 (-0.4307, -37) -> (-4.7608, -34.5)
  line L448 (-4.7608, -34.5) -> (-9.0909, -37)
  line L449 (-9.0909, -37) -> (-9.0909, -42)
  line L450 (-9.0909, -42) -> (-4.7608, -44.5)
  line L451 (-4.7608, -44.5) -> (-0.4307, -42)
  line L452 (-12.3398, -42) -> (-12.3398, -37)
  line L453 (-12.3398, -37) -> (-16.6699, -34.5)
  line L454 (-16.6699, -34.5) -> (-21, -37)
  line L455 (-21, -37) -> (-21, -42)
  line L456 (-21, -42) -> (-16.6699, -44.5)
  line L457 (-16.6699, -44.5) -> (-12.3398, -42)
  line L458 (-24.2488, -42) -> (-24.2488, -37)
  line L459 (-24.2488, -37) -> (-28.579, -34.5)
  line L460 (-28.579, -34.5) -> (-32.9091, -37)
  line L461 (-32.9091, -37) -> (-32.9091, -42)
  line L462 (-32.9091, -42) -> (-28.579, -44.5)
  line L463 (-28.579, -44.5) -> (-24.2488, -42)
  line L464 (-36.1579, -42) -> (-36.1579, -37)
  line L465 (-36.1579, -37) -> (-40.4881, -34.5)
  line L466 (-40.4881, -34.5) -> (-44.8182, -37)
  line L467 (-44.8182, -37) -> (-44.8182, -42)
  line L468 (-44.8182, -42) -> (-40.4881, -44.5)
  line L469 (-40.4881, -44.5) -> (-36.1579, -42)
  line L470 (-48.067, -42) -> (-48.067, -37)
  line L471 (-48.067, -37) -> (-52.3972, -34.5)
  line L472 (-52.3972, -34.5) -> (-56.7273, -37)
  line L473 (-56.7273, -37) -> (-56.7273, -42)
  line L474 (-56.7273, -42) -> (-52.3972, -44.5)
  line L475 (-52.3972, -44.5) -> (-48.067, -42)
  line L476 (-59.9761, -42) -> (-59.9761, -37)
  line L477 (-59.9761, -37) -> (-64.3062, -34.5)
  line L478 (-64.3062, -34.5) -> (-68.6364, -37)
  line L479 (-68.6364, -37) -> (-68.6364, -42)
  line L480 (-68.6364, -42) -> (-64.3062, -44.5)
  line L481 (-64.3062, -44.5) -> (-59.9761, -42)
  line L482 (-71.8852, -42) -> (-71.8852, -37)
  line L483 (-71.8852, -37) -> (-76.2153, -34.5)
  line L484 (-76.2153, -34.5) -> (-80.5455, -37)
  line L485 (-80.5455, -37) -> (-80.5455, -42)
  line L486 (-80.5455, -42) -> (-76.2153, -44.5)
  line L487 (-76.2153, -44.5) -> (-71.8852, -42)
  line L488 (-83.7943, -42) -> (-83.7943, -37)
  line L489 (-83.7943, -37) -> (-88.1244, -34.5)
  line L490 (-88.1244, -34.5) -> (-92.4546, -37)
  line L491 (-92.4546, -37) -> (-92.4546, -42)
  line L492 (-92.4546, -42) -> (-88.1244, -44.5)
  line L493 (-88.1244, -44.5) -> (-83.7943, -42)
  line L494 (-95.7034, -42) -> (-95.7034, -37)
  line L495 (-95.7034, -37) -> (-100.0335, -34.5)
  line L496 (-100.0335, -34.5) -> (-104.3636, -37)
  line L497 (-104.3636, -37) -> (-104.3636, -42)
  line L498 (-104.3636, -42) -> (-100.0335, -44.5)
  line L499 (-100.0335, -44.5) -> (-95.7034, -42)
  line L500 (-107.6125, -42) -> (-107.6125, -37)
  line L501 (-107.6125, -37) -> (-111.9426, -34.5)
  line L502 (-111.9426, -34.5) -> (-116.2727, -37)
  line L503 (-116.2727, -37) -> (-116.2727, -42)
  line L504 (-116.2727, -42) -> (-111.9426, -44.5)
  line L505 (-111.9426, -44.5) -> (-107.6125, -42)
  line L506 (-119.5216, -42) -> (-119.5216, -37)
  line L507 (-119.5216, -37) -> (-123.8517, -34.5)
  line L508 (-123.8517, -34.5) -> (-128.1818, -37)
  line L509 (-128.1818, -37) -> (-128.1818, -42)
  line L510 (-128.1818, -42) -> (-123.8517, -44.5)
  line L511 (-123.8517, -44.5) -> (-119.5216, -42)
  line L512 (-131.4307, -42) -> (-131.4307, -37)
  line L513 (-131.4307, -37) -> (-135.7608, -34.5)
  line L514 (-135.7608, -34.5) -> (-140.0909, -37)
  line L515 (-140.0909, -37) -> (-140.0909, -42)
  line L516 (-140.0909, -42) -> (-135.7608, -44.5)
  line L517 (-135.7608, -44.5) -> (-131.4307, -42)
  line L518 (-19.0502, -52.75) -> (-19.0502, -47.75)
  line L519 (-19.0502, -47.75) -> (-23.3803, -45.25)
  line L520 (-23.3803, -45.25) -> (-27.7105, -47.75)
  line L521 (-27.7105, -47.75) -> (-27.7105, -52.75)
  line L522 (-27.7105, -52.75) -> (-23.3803, -55.25)
  line L523 (-23.3803, -55.25) -> (-19.0502, -52.75)
  line L524 (-30.9593, -52.75) -> (-30.9593, -47.75)
  line L525 (-30.9593, -47.75) -> (-35.2894, -45.25)
  line L526 (-35.2894, -45.25) -> (-39.6196, -47.75)
  line L527 (-39.6196, -47.75) -> (-39.6196, -52.75)
  line L528 (-39.6196, -52.75) -> (-35.2894, -55.25)
  line L529 (-35.2894, -55.25) -> (-30.9593, -52.75)
  line L530 (-42.8684, -52.75) -> (-42.8684, -47.75)
  line L531 (-42.8684, -47.75) -> (-47.1985, -45.25)
  line L532 (-47.1985, -45.25) -> (-51.5286, -47.75)
  line L533 (-51.5286, -47.75) -> (-51.5286, -52.75)
  line L534 (-51.5286, -52.75) -> (-47.1985, -55.25)
  line L535 (-47.1985, -55.25) -> (-42.8684, -52.75)
  line L536 (-54.7775, -52.75) -> (-54.7775, -47.75)
  line L537 (-54.7775, -47.75) -> (-59.1076, -45.25)
  line L538 (-59.1076, -45.25) -> (-63.4377, -47.75)
  line L539 (-63.4377, -47.75) -> (-63.4377, -52.75)
  line L540 (-63.4377, -52.75) -> (-59.1076, -55.25)
  line L541 (-59.1076, -55.25) -> (-54.7775, -52.75)
  line L542 (-66.6866, -52.75) -> (-66.6866, -47.75)
  line L543 (-66.6866, -47.75) -> (-71.0167, -45.25)
  line L544 (-71.0167, -45.25) -> (-75.3468, -47.75)
  line L545 (-75.3468, -47.75) -> (-75.3468, -52.75)
  line L546 (-75.3468, -52.75) -> (-71.0167, -55.25)
  line L547 (-71.0167, -55.25) -> (-66.6866, -52.75)
  line L548 (-78.5957, -52.75) -> (-78.5957, -47.75)
  line L549 (-78.5957, -47.75) -> (-82.9258, -45.25)
  line L550 (-82.9258, -45.25) -> (-87.2559, -47.75)
  line L551 (-87.2559, -47.75) -> (-87.2559, -52.75)
  line L552 (-87.2559, -52.75) -> (-82.9258, -55.25)
  line L553 (-82.9258, -55.25) -> (-78.5957, -52.75)
  line L554 (-90.5048, -52.75) -> (-90.5048, -47.75)
  line L555 (-90.5048, -47.75) -> (-94.8349, -45.25)
  line L556 (-94.8349, -45.25) -> (-99.165, -47.75)
  line L557 (-99.165, -47.75) -> (-99.165, -52.75)
  line L558 (-99.165, -52.75) -> (-94.8349, -55.25)
  line L559 (-94.8349, -55.25) -> (-90.5048, -52.75)
  line L560 (-102.4138, -52.75) -> (-102.4138, -47.75)
  line L561 (-102.4138, -47.75) -> (-106.744, -45.25)
  line L562 (-106.744, -45.25) -> (-111.0741, -47.75)
  line L563 (-111.0741, -47.75) -> (-111.0741, -52.75)
  line L564 (-111.0741, -52.75) -> (-106.744, -55.25)
  line L565 (-106.744, -55.25) -> (-102.4138, -52.75)
  line L566 (-114.3229, -52.75) -> (-114.3229, -47.75)
  line L567 (-114.3229, -47.75) -> (-118.6531, -45.25)
  line L568 (-118.6531, -45.25) -> (-122.9832, -47.75)
  line L569 (-122.9832, -47.75) -> (-122.9832, -52.75)
  line L570 (-122.9832, -52.75) -> (-118.6531, -55.25)
  line L571 (-118.6531, -55.25) -> (-114.3229, -52.75)
  line L572 (-126.232, -52.75) -> (-126.232, -47.75)
  line L573 (-126.232, -47.75) -> (-130.5622, -45.25)
  line L574 (-130.5622, -45.25) -> (-134.8923, -47.75)
  line L575 (-134.8923, -47.75) -> (-134.8923, -52.75)
  line L576 (-134.8923, -52.75) -> (-130.5622, -55.25)
  line L577 (-130.5622, -55.25) -> (-126.232, -52.75)
  line L578 (-138.1411, -52.75) -> (-138.1411, -47.75)
  line L579 (-138.1411, -47.75) -> (-142.4712, -45.25)
  line L580 (-142.4712, -45.25) -> (-146.8014, -47.75)
  line L581 (-146.8014, -47.75) -> (-146.8014, -52.75)
  line L582 (-146.8014, -52.75) -> (-142.4712, -55.25)
  line L583 (-142.4712, -55.25) -> (-138.1411, -52.75)
  line L584 (-150.0502, -52.75) -> (-150.0502, -47.75)
  line L585 (-150.0502, -47.75) -> (-154.3803, -45.25)
  line L586 (-154.3803, -45.25) -> (-158.7105, -47.75)
  line L587 (-158.7105, -47.75) -> (-158.7105, -52.75)
  line L588 (-158.7105, -52.75) -> (-154.3803, -55.25)
  line L589 (-154.3803, -55.25) -> (-150.0502, -52.75)
  line L590 (-37.6698, -63.5) -> (-37.6698, -58.5)
  line L591 (-37.6698, -58.5) -> (-41.9999, -56)
  line L592 (-41.9999, -56) -> (-46.33, -58.5)
  line L593 (-46.33, -58.5) -> (-46.33, -63.5)
  line L594 (-46.33, -63.5) -> (-41.9999, -66)
  line L595 (-41.9999, -66) -> (-37.6698, -63.5)
  line L596 (-49.5788, -63.5) -> (-49.5788, -58.5)
  line L597 (-49.5788, -58.5) -> (-53.909, -56)
  line L598 (-53.909, -56) -> (-58.2391, -58.5)
  line L599 (-58.2391, -58.5) -> (-58.2391, -63.5)
  line L600 (-58.2391, -63.5) -> (-53.909, -66)
  line L601 (-53.909, -66) -> (-49.5788, -63.5)
  line L602 (-61.4879, -63.5) -> (-61.4879, -58.5)
  line L603 (-61.4879, -58.5) -> (-65.8181, -56)
  line L604 (-65.8181, -56) -> (-70.1482, -58.5)
  line L605 (-70.1482, -58.5) -> (-70.1482, -63.5)
  line L606 (-70.1482, -63.5) -> (-65.8181, -66)
  line L607 (-65.8181, -66) -> (-61.4879, -63.5)
  line L608 (-73.397, -63.5) -> (-73.397, -58.5)
  line L609 (-73.397, -58.5) -> (-77.7272, -56)
  line L610 (-77.7272, -56) -> (-82.0573, -58.5)
  line L611 (-82.0573, -58.5) -> (-82.0573, -63.5)
  line L612 (-82.0573, -63.5) -> (-77.7272, -66)
  line L613 (-77.7272, -66) -> (-73.397, -63.5)
  line L614 (-85.3061, -63.5) -> (-85.3061, -58.5)
  line L615 (-85.3061, -58.5) -> (-89.6362, -56)
  line L616 (-89.6362, -56) -> (-93.9664, -58.5)
  line L617 (-93.9664, -58.5) -> (-93.9664, -63.5)
  line L618 (-93.9664, -63.5) -> (-89.6362, -66)
  line L619 (-89.6362, -66) -> (-85.3061, -63.5)
  line L620 (-97.2152, -63.5) -> (-97.2152, -58.5)
  line L621 (-97.2152, -58.5) -> (-101.5453, -56)
  line L622 (-101.5453, -56) -> (-105.8755, -58.5)
  line L623 (-105.8755, -58.5) -> (-105.8755, -63.5)
  line L624 (-105.8755, -63.5) -> (-101.5453, -66)
  line L625 (-101.5453, -66) -> (-97.2152, -63.5)
  line L626 (-109.1243, -63.5) -> (-109.1243, -58.5)
  line L627 (-109.1243, -58.5) -> (-113.4544, -56)
  line L628 (-113.4544, -56) -> (-117.7846, -58.5)
  line L629 (-117.7846, -58.5) -> (-117.7846, -63.5)
  line L630 (-117.7846, -63.5) -> (-113.4544, -66)
  line L631 (-113.4544, -66) -> (-109.1243, -63.5)
  line L632 (-121.0334, -63.5) -> (-121.0334, -58.5)
  line L633 (-121.0334, -58.5) -> (-125.3635, -56)
  line L634 (-125.3635, -56) -> (-129.6936, -58.5)
  line L635 (-129.6936, -58.5) -> (-129.6936, -63.5)
  line L636 (-129.6936, -63.5) -> (-125.3635, -66)
  line L637 (-125.3635, -66) -> (-121.0334, -63.5)
  line L638 (-132.9425, -63.5) -> (-132.9425, -58.5)
  line L639 (-132.9425, -58.5) -> (-137.2726, -56)
  line L640 (-137.2726, -56) -> (-141.6027, -58.5)
  line L641 (-141.6027, -58.5) -> (-141.6027, -63.5)
  line L642 (-141.6027, -63.5) -> (-137.2726, -66)
  line L643 (-137.2726, -66) -> (-132.9425, -63.5)
  line L644 (-144.8516, -63.5) -> (-144.8516, -58.5)
  line L645 (-144.8516, -58.5) -> (-149.1817, -56)
  line L646 (-149.1817, -56) -> (-153.5118, -58.5)
  line L647 (-153.5118, -58.5) -> (-153.5118, -63.5)
  line L648 (-153.5118, -63.5) -> (-149.1817, -66)
  line L649 (-149.1817, -66) -> (-144.8516, -63.5)
  line L650 (-156.7607, -63.5) -> (-156.7607, -58.5)
  line L651 (-156.7607, -58.5) -> (-161.0908, -56)
  line L652 (-161.0908, -56) -> (-165.4209, -58.5)
  line L653 (-165.4209, -58.5) -> (-165.4209, -63.5)
  line L654 (-165.4209, -63.5) -> (-161.0908, -66)
  line L655 (-161.0908, -66) -> (-156.7607, -63.5)
  line L656 (-168.6698, -63.5) -> (-168.6698, -58.5)
  line L657 (-168.6698, -58.5) -> (-172.9999, -56)
  line L658 (-172.9999, -56) -> (-177.33, -58.5)
  line L659 (-177.33, -58.5) -> (-177.33, -63.5)
  line L660 (-177.33, -63.5) -> (-172.9999, -66)
  line L661 (-172.9999, -66) -> (-168.6698, -63.5)
  point P0 (-33.9385, -16.7046)
  point P1 (106.9565, 25)
  dimension "d46" = 5
  dimension "d49" = 131
  dimension "d50" = 172
  constraint tangent L8 A0
  constraint tangent A0 L9
  constraint parallel L8 L9
  constraint tangent L9 A1
  constraint tangent L8 A1
  constraint horizontal L10
  constraint midpoint L10 P0
  constraint horizontal L19
  measures "d46" distance of L13.start P1
extrude "Extrusion13" cut sketch "Skizze9" against normal blind 90 contours A1 L410 L411 L412 | L8 L404 L405 L406 L407 | A1 L350 L351 L352 L354 L355 | L8 L398 L399 L400 L401 | A1 L284 L285 L287 L288 L289 | L8 L392 L393 L394 L395 | L9 L278 L279 L280 L281 L282 L283 | A0 L387 L388 L389 | L9 L272 L273 L274 L275 L276 L277 | A0 L322 L323 L324 | L9 L266 L267 L268 L269 L270 L271 | A0 L262 L263 L264 L265 | L326 L327 L328 L329 L330 L331 | L332 L333 L334 L335 L336 L337 | L338 L339 L340 L341 L342 L343 | L344 L345 L346 L347 L348 L349 bodies 2
sketch "Skizze10" plane through (0, 0, -33) normal (0, 0, -1) x (1, 0, 0)
  line L0 (-2, -15.5) -> (-0.5, -15.5)
  line L1 (-0.5, -15.5) -> (-0.5, 0.5)
  line L2 (-0.5, 0.5) -> (77.5, 0.5)
  line L3 (77.5, 0.5) -> (77.5, -50)
  line L4 (77.5, -50) -> (-0.5, -50)
  line L5 (-0.5, -50) -> (-0.5, -21.5)
  line L6 (-0.5, -21.5) -> (-2, -21.5)
  line L7 (-2, -21.5) -> (-2, -51.5)
  line L8 (-2, -51.5) -> (79, -51.5)
  line L9 (79, -51.5) -> (79, 2)
  line L10 (79, 2) -> (-2, 2)
  line L11 (-2, 2) -> (-2, -15.5)
  line L12 (-2, -21.5) -> (-3.8, -21.5)
  line L13 (-3.8, -21.5) -> (-3.8, -24.5)
  line L14 (-3.8, -24.5) -> (-2, -24.5)
  line L15 (-2, -24.5) -> (-2, -21.5)
  line L16 (-2, -15.5) -> (-3.8, -15.5)
  line L17 (-3.8, -15.5) -> (-3.8, -12.5)
  line L18 (-3.8, -12.5) -> (-2, -12.5)
  line L19 (-2, -12.5) -> (-2, -15.5)
  line L20 (-3.8, -24.5) -> (-5.3, -24.5)
  line L21 (-5.3, -24.5) -> (-5.3, -12.5)
  line L22 (-5.3, -12.5) -> (-3.8, -12.5)
  line L23 (-3.8, -12.5) -> (-3.8, -24.5)
  line L24 (-5.3, -24.5) -> (-2, -24.5)
  line L25 (-2, -24.5) -> (-2, -26)
  line L26 (-2, -26) -> (-5.3, -26)
  line L27 (-5.3, -26) -> (-5.3, -24.5)
  line L28 (-5.3, -12.5) -> (-2, -12.5)
  line L29 (-2, -12.5) -> (-2, -11)
  line L30 (-2, -11) -> (-5.3, -11)
  line L31 (-5.3, -11) -> (-5.3, -12.5)
  dimension "d53" = 1.8
  dimension "d54" = 3
  dimension "d55" = 1.8
  dimension "d56" = 3
  dimension "d57" = 1.5
  dimension "d58" = 1.5
  constraint horizontal L12
  constraint vertical L13
  constraint horizontal L14
  constraint vertical L15
  constraint coincident L6.end L7.start
  constraint horizontal L16
  constraint vertical L17
  constraint horizontal L18
  constraint vertical L19
  constraint coincident L0.start L11.end
  constraint horizontal L20
  constraint vertical L21
  constraint horizontal L22
  constraint vertical L23
  constraint horizontal L24
  constraint vertical L25
  constraint horizontal L26
  constraint vertical L27
  constraint coincident L7 L25.end
  constraint horizontal L28
  constraint vertical L29
  constraint horizontal L30
  constraint vertical L31
  constraint coincident L11 L29.end
  measures "d53" distance of L6.end L12.end
  measures "d54" distance of L6.end L14.end
  measures "d55" distance of L0.start L16.end
  measures "d56" distance of L0.start L18.end
  measures "d57" distance of L13.end L20.end
  measures "d58" distance of L21.end L30.end
extrude "Extrusion14" add sketch "Skizze10" against normal blind 35 contours L11 L18 L22 L28 L29 L30 L31 | L13 L17 L20 L21 L22 L23 L24 L28 | L7 L14 L20 L24 L25 L26 L27 bodies 2
sketch "Skizze11" plane through (-5.3, 0, 0) normal (-1, 0, 0) x (0, -1, 0)
  line L0 (-26, -33) -> (-11, -33)
  line L1 (-11, -33) -> (-11, 2)
  line L2 (-11, 2) -> (-26, 2)
  line L3 (-26, 2) -> (-26, -33)
  arc A0 (-15.5268, -6) -> (-21.4732, -6) centre (-18.5, -6.4) ccw
  circle A1 centre (-18.5, -6.4) radius 3
  line L4 (-15.5, -33) -> (-15.5, -6)
  line L5 (-21.5, -6) -> (-21.5, -33)
  constraint concentric A0 A1
  constraint coincident A0.end A1
extrude "Extrusion15" cut sketch "Skizze11" against normal blind 5 contours L0 A1 L4 L5 | A0 A1 bodies 2
sketch "Skizze12" plane through (0, 0, 2) normal (0, 0, 1) x (-1, 0, 0)
  line L0 (2, -11) -> (2, 2)
  line L1 (2, 2) -> (-79, 2)
  line L2 (-79, 2) -> (-79, -51.5)
  line L3 (-79, -51.5) -> (2, -51.5)
  line L4 (2, -51.5) -> (2, -26)
  line L5 (2, -26) -> (5.3, -26)
  line L6 (5.3, -26) -> (5.3, -11)
  line L7 (5.3, -11) -> (2, -11)
  line L8 (2, -12.5) -> (3.8, -12.5)
  line L9 (3.8, -12.5) -> (3.8, -24.5)
  line L10 (3.8, -24.5) -> (2, -24.5)
  line L11 (2, -24.5) -> (2, -12.5)
extrude "Extrusion16" add sketch "Skizze12" against normal blind 5.4 contours L8 L9 L10 L11 bodies 2
sketch "Skizze13" plane through (0, 0, -3.4) normal (0, 0, -1) x (1, 0, 0)
  line L0 (-3.8, -24.5) -> (-2, -24.5)
  line L1 (-2, -24.5) -> (-2, -18.5)
  line L2 (-2, -18.5) -> (-2, -12.5)
  line L3 (-2, -12.5) -> (-3.8, -12.5)
  line L4 (-3.8, -12.5) -> (-3.8, -18.5)
  line L5 (-3.8, -18.5) -> (-3.8, -24.5)
  line L6 (-2.2, -18.5) -> (-2.2, -12.7)
  line L7 (-2.2, -12.7) -> (-3.6, -12.7)
  line L8 (-3.6, -12.7) -> (-3.6, -18.5)
  line L9 (-3.6, -18.5) -> (-3.6, -24.3)
  line L10 (-3.6, -24.3) -> (-2.2, -24.3)
  line L11 (-2.2, -24.3) -> (-2.2, -18.5)
  dimension "d65" = -0.2
extrude "Extrusion17" add sketch "Skizze13" along normal blind 29.4 from surface at 0.2 separate body contours L6 L7 L8 L9 L10 L11 makes body 3
extrude "Extrusion18" cut sketch "Skizze11" against normal blind 6 contours A0 A1 bodies 3
sketch "Skizze14" plane through (-3.6, 0, 0) normal (-1, 0, 0) x (0, -1, 0)
  arc A0 (-19.577, -3.6) -> (-17.423, -3.6) centre (-18.5, -6.4) ccw
  line L0 (-19.577, -3.6) -> (-24.3, -3.6)
  line L1 (-24.3, -3.6) -> (-24.3, -33)
  line L2 (-24.3, -33) -> (-12.7, -33)
  line L3 (-12.7, -33) -> (-12.7, -3.6)
  line L4 (-12.7, -3.6) -> (-17.423, -3.6)
  line L5 (-21.5, -11.6495) -> (-21.5, -3.1345)
  line L6 (-15.5, -11.334) -> (-15.5, -3.6)
  arc A1 (-19.577, -3.6) -> (-17.423, -3.6) centre (-18.5, -6.4) ccw
  constraint coincident L4 L6.end
  constraint perpendicular L4 L6
  constraint tangent A0 L6
  constraint tangent A0 L5
  constraint vertical L5
extrude "Extrusion19" cut sketch "Skizze14" against normal blind 3 contours A0 L0 L5 A1 | A0 L4 L6 A1 bodies 3